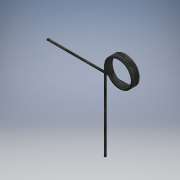
# Autodesk Inventor part: TOS 0.3-4-270ﾟ-3
Saved by Autodesk Inventor 2017 (Build 210142000, 142)
## iProperties
Part Number: TOS 0.3-4-270ﾟ-3
Material: 鋼
Document SubType Name: Modeling
Designer: sktom
Density: 7.85 g/cm^3
Appearance: プレート
Author: sktom
Autodesk Inventor part; units mm, degrees
ref_plane "YZ Plane" through (0, 0, 0) normal (1, 0, 0) x (0, 1, 0)
ref_plane "XZ Plane" through (0, 0, 0) normal (0, 1, 0) x (-1, 0, 0)
ref_plane "XY Plane" through (0, 0, 0) normal (0, 0, 1) x (1, 0, 0)
sketch "スケッチ1" plane through (0, 0, 0) normal (0, 0, 1) x (1, 0, 0)
  circle A0 centre (-2, 0) radius 0.15
  point P0 (0, 0)
  dimension "d0" = 0.3
  dimension "d1" = 2
  constraints: 1 centre point, 1 horizontal alignment
  measures "d0" diameter of A0
  measures "d1" distance of point (0, 0) A0.centre
coil "コイル1" sketch "スケッチ1" operation add axis through (0, -10, 0) along (0, 1, 0) pitch 0.31 turns 3.75 hand right
sketch "スケッチ2" plane through (-2, 0, 0) normal (0, 0, -1) x (-1, 0, 0)
  circle A0 centre (0, 0) radius 0.15 projected
  point P0 (-2, 0)
  point P1 (-0.15, 0)
  constraints: 1 horizontal alignment
extrude "押し出し1" add sketch "スケッチ2" along normal blind 12
sketch "スケッチ3" plane through (0, 1.1625, -2) normal (-1, 0, 0) x (0, 0, 1)
  circle A0 centre (0, 0) radius 0.15 projected
  point P0 (2, -1.1625)
  point P1 (0.15, 0)
  constraints: 1 horizontal alignment
extrude "押し出し2" add sketch "スケッチ3" along normal blind 12
